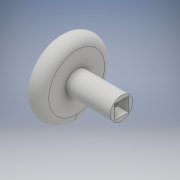
# Autodesk Inventor part: joystick_nibble
Saved by Autodesk Inventor 2018 (Build 220112000, 112)
## iProperties
Created: 2018-03-13
Part Number: joystick_nibble
Material: Generic
Document SubType Name: Modeling
Designer: oechslin
Density: 1 g/cm^3
Appearance: Default
Author: oechslin
Autodesk Inventor part; units mm, degrees
ref_plane "YZ Plane" through (0, 0, 0) normal (1, 0, 0) x (0, 1, 0)
ref_plane "XZ Plane" through (0, 0, 0) normal (0, 1, 0) x (-1, 0, 0)
ref_plane "XY Plane" through (0, 0, 0) normal (0, 0, 1) x (1, 0, 0)
sketch "Sketch1" plane through (0, 0, 0) normal (0, 1, 0) x (-1, 0, 0)
  line L0 (3.9616, 0) -> (-12.9611, 0)
  line L1 (-12.9611, 0) -> (-12.9611, -3)
  line L2 (-12.9611, -3) -> (-0.9611, -3)
  line L3 (-12.9611, -3) -> (-0.9611, -3) construction
  line L4 (-0.9611, -3) -> (-0.9611, -11.5)
  line L5 (-0.9611, -11.5) -> (3.0389, -11.5)
  arc A0 (3.0389, -11.5) -> (3.9616, 0) centre (-48.7312, -1.5591) ccw
  line L6 (61.7439, 0) -> (-67.1437, 0) projected
  arc A1 (3.3616, 0) -> (3.8723, -5) centre (43.3314, 1.556) ccw
  line L7 (3.8723, -5) -> (7.1647, 0)
  line L8 (7.1647, 0) -> (3.3616, 0)
  point P0 (0, 0)
  dimension "d1" = 3
  dimension "d2" = 90
  dimension "d3" = 12
  dimension "d5" = 8.5
  dimension "d6" = 4
  dimension "d11" = 0
  dimension "d14" = 0.6
  dimension "d16" = 5
  dimension "d17" = 40
  constraints: 16 end point, 5 point on circle, 4 horizontal, 2 centre point, 2 collinear, 2 perpendicular, 2 point on line
  measures "d1" distance of L0.end L1.end
  measures "d2" angle of L1 L0
  measures "d3" distance of L1.end L2.end
  measures "d5" distance of L2.end L4.end
  measures "d6" distance of L4.end L5.end
  measures "d11" distance between parallel lines of L0 L6
  measures "d14" distance of L8.end L0.start
  measures "d16" distance from line of L6 L7.start
  measures "d17" radius of A1
revolve "Revolution1" add sketch "Sketch1" angle 360 about axis through (-10, 0, 0) along (1, 0, 0) contours A0 A1 L0 | A1 A0 L5 L4 L2 L1 L0
fillet "Fillet1" radius 2.3 2 edges at (-3.0389, 0, 11.5) (0.9611, 0, 11.5)
sketch "Sketch2" plane through (12.9611, 0, 0) normal (1, 0, 0) x (0, 0, -1)
  circle A0 centre (0, 0) radius 3 projected
  line L0 (1.9, 1.9) -> (-1.9, 1.9)
  line L1 (-1.9, 1.9) -> (-1.9, -1.9)
  line L2 (-1.9, -1.9) -> (1.9, -1.9)
  line L3 (1.9, -1.9) -> (1.9, 1.9)
  line L4 (1.9, 1.9) -> (-1.9, -1.9) construction
  line L5 (-1.9, 1.9) -> (1.9, -1.9) construction
  dimension "d9" = 3.8
  dimension "d10" = 3.8
  constraints: 12 end point, 2 midpoint, 2 parallel, 1 horizontal, 1 perpendicular
  measures "d9" distance of L2.end L1.end
  measures "d10" distance of L1.end L0.end
extrude "Extrusion1" cut sketch "Sketch2" against normal blind 3 contours L3 L2 L1 L0
revolve "Revolution2" cut sketch "Sketch1" angle 360 about axis through (-10, 0, 0) along (1, 0, 0) contours A0 A1 L0 | L6 L7 A0
body "Solid1"
